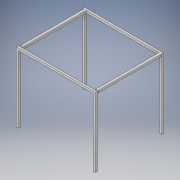
# Autodesk Inventor part: MetalTable
Saved by Autodesk Inventor 2019 (Build 230136000, 136)
## iProperties
Created: 2018-05-11
Part Number: MetalTable
Material: Generic
Document SubType Name: Modeling
Designer: steele
Density: 1 g/cm^3
Appearance: Default
Author: steele
Autodesk Inventor part; units mm, degrees
ref_plane "YZ Plane" through (0, 0, 0) normal (1, 0, 0) x (0, 1, 0)
sketch "Sketch3" plane through (0, 0, 0) normal (0, 1, 0) x (-1, 0, 0)
  line L0 (6.35, 6.2855) -> (-6.35, 6.2855)
  line L1 (-6.35, 6.2855) -> (-6.35, -6.2855)
  line L2 (-6.35, -6.2855) -> (6.35, -6.2855)
  line L3 (6.35, -6.2855) -> (6.35, 6.2855)
  line L4 (6.35, 6.2855) -> (-6.35, -6.2855) construction
  line L5 (-6.35, 6.2855) -> (6.35, -6.2855) construction
  point P0 (0, 0)
  dimension "d7" = 12.7
  constraints: 12 end point, 2 midpoint, 2 parallel, 1 horizontal, 1 perpendicular
  measures "d7" distance of L0.start L0.end
sketch3d "3D Sketch1"
  line L0 (0, 0, 0) -> (0, 406.4, 0)
  line L1 (0, 406.4, 0) -> (457.2, 406.4, 0)
  line L2 (457.2, 406.4, 0) -> (457.2, 0, 0)
  dimension "d0" = 406.4
  dimension "d1" = 457.2
  dimension "d2" = 457.2
  dimension "d3" = 406.4
  dimension "d4" = 406.4
  dimension "d5" = 406.4
  dimension "d6" = 406.4
sweep "Sweep3" add profiles "Sketch3" path "3D Sketch1"
ref_plane "Work Plane1" through (-6.35, 412.75, -196.9145) normal (0, 0, 1) x (1, 0, 0)
mirror "Mirror1" about plane through (-6.35, 412.75, -196.9145) normal (0, 0, 1) of "Sweep3"
sketch "Sketch4" plane through (-6.35, 412.75, -387.5435) normal (0, 0, 1) x (1, 0, 0)
  line L0 (453.1353, -12.5225) -> (468.8842, -12.5225)
  line L1 (468.8842, -12.5225) -> (468.8842, 0)
  line L2 (468.8842, 0) -> (453.1353, 0)
  line L3 (453.1353, 0) -> (453.1353, -12.5225)
  line L4 (453.1353, -12.5225) -> (468.8842, 0) construction
  line L5 (468.8842, -12.5225) -> (453.1353, 0) construction
  point P0 (6.35, -412.75)
  point P1 (461.0098, -6.2613)
  constraints: 12 end point, 2 midpoint, 2 parallel, 1 horizontal, 1 perpendicular
sketch3d "3D Sketch2"
  line L0 (457.2, 406.4, -384.0365) -> (457.2, 406.4, -8.0315)
sweep "Sweep4" add profiles "Sketch4" path "3D Sketch2"
ref_plane "Work Plane2" through (230.8853, 400.2275, -387.5435) normal (-1, 0, 0) x (0, 0, 1)
mirror "Mirror2" about plane through (230.8853, 400.2275, -387.5435) normal (-1, 0, 0) of "Sweep4"
body "Solid3"
